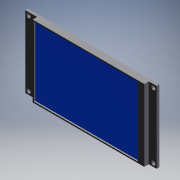
# Autodesk Inventor part: NextionDisplay
Saved by Autodesk Inventor 2019 (Build 230136000, 136)
## iProperties
Created: 2020-10-19
Part Number: NextionDisplay
Material: Типовые
Document SubType Name: Modeling
Designer: Surflay
Density: 1 g/cm^3
Appearance: По умолчанию
Author: Surflay
Autodesk Inventor part; units mm, degrees
ref_plane "YZ Plane" through (0, 0, 0) normal (1, 0, 0) x (0, 1, 0)
ref_plane "XZ Plane" through (0, 0, 0) normal (0, 1, 0) x (-1, 0, 0)
ref_plane "XY Plane" through (0, 0, 0) normal (0, 0, 1) x (1, 0, 0)
sketch "Эскиз1" plane through (0, 0, 0) normal (0, 0, 1) x (1, 0, 0)
  line L0 (0, 0) -> (100.5, 0)
  line L1 (100.5, 0) -> (100.5, 54.94)
  line L2 (100.5, 54.94) -> (0, 54.94)
  line L3 (0, 54.94) -> (0, 0)
  circle A0 centre (2.5, 52.44) radius 1.5
  circle A1 centre (98, 52.44) radius 1.5
  line L4 (196, 54.94) -> (95.5, 54.94)
  circle A2 centre (2.5, 2.5) radius 1.5
  circle A3 centre (98, 2.5) radius 1.5
  dimension "d0" = 100.5
  dimension "d1" = 54.94
  dimension "d2" = 3
  dimension "d3" = 2.5
  dimension "d4" = 2.5
  dimension "d7" = 95.5
  dimension "d14" = 49.94
  constraints: 10 end point, 4 centre point, 2 horizontal, 2 parallel, 1 collinear, 1 perpendicular, 1 vertical, 8 other
  measures "d0" distance of L2.end L1.end
  measures "d1" distance of L1.end L0.end
  measures "d2" diameter of A0
  measures "d3" distance from line of L2 A0.centre
  measures "d4" distance from line of L3 A0.centre
  measures "d7" distance of A0.centre A1.centre
  measures "d14" distance of A0.centre A2.centre
extrude "Выдавливание1" add sketch "Эскиз1" along normal blind 5.45
sketch "Эскиз2" plane through (0, 0, 5.45) normal (0, 0, 1) x (1, 0, 0)
  line L0 (9, 54.94) -> (94.5, 54.94)
  line L1 (94.5, 54.94) -> (94.5, 0)
  line L2 (94.5, 0) -> (9, 0)
  line L3 (9, 0) -> (9, 54.94)
  line L4 (100.5, 54.94) -> (0, 54.94) projected
  line L5 (100.5, 0) -> (100.5, 54.94) projected
  line L6 (-12, 65) -> (119, 65)
  line L7 (119, 65) -> (119, -14)
  line L8 (119, -14) -> (-12, -14)
  line L9 (-12, -14) -> (-12, 65)
  point P0 (0, 0)
  point P1 (50.25, 54.94)
  dimension "d21" = 85.5
  dimension "d22" = 54.94
  dimension "d23" = 6
  constraints: 16 end point, 4 parallel, 2 horizontal, 2 perpendicular, 1 midpoint, 1 point on line
  measures "d21" distance of L1.end L2.end
  measures "d22" distance of L0.end L1.end
  measures "d23" distance between parallel lines of L5 L1
extrude "Выдавливание2" cut sketch "Эскиз2" against normal blind 3.45
sketch "Эскиз3" plane through (0, 0, 5.45) normal (0, 0, 1) x (1, 0, 0)
  line L0 (10, 53.94) -> (89.5, 53.94)
  line L1 (89.5, 53.94) -> (89.5, 1)
  line L2 (89.5, 1) -> (10, 1)
  line L3 (10, 1) -> (10, 53.94)
  line L4 (94.5, 54.94) -> (9, 54.94) projected
  line L5 (9, 54.94) -> (9, 0) projected
  line L6 (9, 0) -> (94.5, 0) projected
  line L7 (94.5, 0) -> (94.5, 54.94) projected
  point P0 (0, 0)
  dimension "d28" = 1
  dimension "d29" = 1
  dimension "d30" = 1
  dimension "d31" = 5
  constraints: 8 end point, 2 parallel, 1 horizontal, 1 perpendicular
  measures "d28" distance between parallel lines of L4 L0
  measures "d29" distance between parallel lines of L5 L3
  measures "d30" distance between parallel lines of L6 L2
  measures "d31" distance between parallel lines of L7 L1
extrude "Выдавливание3" cut sketch "Эскиз3" against normal blind 1 contours L0 L1 L2 L3
